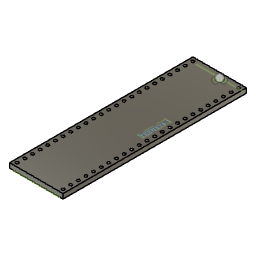
TEENSY4.1PACKAGE v2 (Autodesk Fusion 360 design; units mm, degrees)
Autodesk Fusion 360 part; units mm, degrees
note: some values were not read from the file. Set by a fixed rule: the direction of a hole.
sketch "Sketch1" plane through (0, 0, 0) normal (0, 0, 1) x (1, 0, 0)
  line L0 (0, -1.27) -> (15.24, -1.27)
  line L1 (0, -1.27) -> (15.24, -1.27)
  line L2 (15.24, -1.27) -> (16.51, -1.27)
  line L3 (0, -1.27) -> (-1.27, -1.27)
  line L4 (-1.27, -1.27) -> (16.51, -1.27)
  line L5 (16.51, -1.27) -> (16.51, 59.69)
  line L6 (16.51, 59.69) -> (-1.27, 59.69)
  line L7 (-1.27, 59.69) -> (-1.27, -1.27)
  dimension "d1" = 15.24
  dimension "d2" = 1.27
  dimension "d3" = 1.27
  dimension "d4" = 60.96
  dimension "d5" = 17.78
  constraint horizontal L0
  constraint parallel L0 L2
  constraint coincident L0.start L1.start
  constraint parallel L0 L3
  constraint horizontal L4
  constraint vertical L5
  constraint horizontal L6
  constraint vertical L7
  measures "d1" distance of L0.start L0.end
  measures "d2" distance of L0.end L2.end
  measures "d3" distance of L0.start L3.end
  measures "d4" distance of L3.end L6.end
  measures "d5" distance of L5.end L6.end
extrude "Extrude1" add sketch "Sketch1" along normal blind 1.57
hole "Hole1" at (0, 58.42, 0) at (0, 55.88, 0) at (0, 53.34, 0) at (0, 50.8, 0) at (0, 48.26, 0) at (0, 45.72, 0) at (0, 43.18, 0) at (0, 40.64, 0) at (0, 38.1, 0) at (0, 35.56, 0) at (0, 33.02, 0) at (0, 30.48, 0) at (0, 27.94, 0) at (0, 25.4, 0) at (0, 22.86, 0) at (0, 20.32, 0) at (0, 17.78, 0) at (0, 15.24, 0) at (0, 12.7, 0) at (0, 10.16, 0) at (0, 7.62, 0) at (0, 5.08, 0) at (0, 2.54, 0) at (0, 0, 0) at (15.24, 0, 0) at (15.24, 2.54, 0) at (15.24, 5.08, 0) at (15.24, 7.62, 0) at (15.24, 10.16, 0) at (15.24, 12.7, 0) at (15.24, 15.24, 0) at (15.24, 17.78, 0) at (15.24, 20.32, 0) at (15.24, 22.86, 0) at (15.24, 25.4, 0) at (15.24, 27.94, 0) at (15.24, 30.48, 0) at (15.24, 33.02, 0) at (15.24, 35.56, 0) at (15.24, 38.1, 0) at (15.24, 40.64, 0) at (15.24, 43.18, 0) at (15.24, 45.72, 0) at (15.24, 48.26, 0) at (15.24, 50.8, 0) at (15.24, 53.34, 0) at (15.24, 55.88, 0) at (15.24, 58.42, 0) direction (0, 0, 1) diameter 0.965 depth 1.57 tip angle 180
